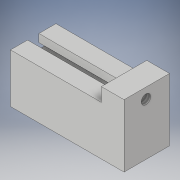
# Autodesk Inventor part: tenshoner base
Saved by Autodesk Inventor 2019 (Build 230136000, 136)
## iProperties
Created: 2019-12-07
Part Number: tenshoner base
Material: Generic
Document SubType Name: Modeling
Designer: User
Density: 1 g/cm^3
Appearance: Default
Author: User
Autodesk Inventor part; units mm, degrees
ref_plane "YZ Plane" through (0, 0, 0) normal (1, 0, 0) x (0, 1, 0)
ref_plane "XZ Plane" through (0, 0, 0) normal (0, 1, 0) x (-1, 0, 0)
ref_plane "XY Plane" through (0, 0, 0) normal (0, 0, 1) x (1, 0, 0)
sketch "Sketch1" plane through (0, 0, 0) normal (1, 0, 0) x (0, 1, 0)
  line L0 (0, 0) -> (13.716, 0)
  line L1 (13.716, 0) -> (13.716, -12.7)
  line L2 (13.716, -12.7) -> (0, -12.7)
  line L3 (0, -12.7) -> (0, 0)
  line L4 (13.716, -4.7625) -> (11.5062, -4.7625)
  line L5 (11.5062, -4.7625) -> (11.5062, -3.175)
  line L6 (11.5062, -3.175) -> (9.906, -3.175)
  line L7 (9.906, -3.175) -> (9.906, -9.525)
  line L8 (9.906, -9.525) -> (11.5062, -9.525)
  line L9 (11.5062, -9.525) -> (11.5062, -7.9375)
  line L10 (11.5062, -7.9375) -> (13.716, -7.9375)
  dimension "d0" = 12.7
  dimension "d1" = 3.175
  dimension "d2" = 6.35
  dimension "d3" = 1.5875
  dimension "d4" = 4.7625
  dimension "d5" = 1.6002
  dimension "d6" = 3.81
  dimension "d7" = 13.716
  constraints: 22 end point, 6 perpendicular, 4 point on line, 2 horizontal, 2 parallel
  measures "d0" distance of L0.end L1.end
  measures "d1" distance between parallel lines of L4 L10
  measures "d2" distance between parallel lines of L8 L6
  measures "d3" distance between parallel lines of L4 L6
  measures "d4" distance between parallel lines of L0 L4
  measures "d5" distance between parallel lines of L7 L5
  measures "d6" distance between parallel lines of L1 L7
  measures "d7" distance between parallel lines of L3 L1
extrude "Extrusion1" add sketch "Sketch1" along normal blind 25.4 contours L0 L1 L4 L5 L6 L7 L8 L9 L10 L2 L3
sketch "Sketch2" plane through (25.4, 0, 0) normal (1, 0, 0) x (0, 0, -1)
  line L0 (0, 0) -> (12.7, 0)
  line L1 (12.7, 0) -> (12.7, 17.526)
  line L2 (12.7, 17.526) -> (0, 17.526)
  line L3 (0, 17.526) -> (0, 0)
  line L4 (12.7, 13.716) -> (7.9375, 13.716) projected
  dimension "d10" = 3.81
  dimension "d11" = 12.7
  constraints: 8 end point, 2 parallel, 1 coincident, 1 horizontal, 1 perpendicular
  measures "d10" distance between parallel lines of L2 L4
  measures "d11" distance between parallel lines of L3 L1
extrude "Extrusion2" add sketch "Sketch2" along normal blind 6.35
sketch "Sketch3" plane through (31.75, 0, 0) normal (1, 0, 0) x (0, 0, -1)
  line L0 (0, 0) -> (12.7, 0) projected
  line L1 (12.7, 0) -> (12.7, 17.526) projected
  line L2 (12.7, 17.526) -> (0, 17.526) projected
  line L3 (0, 17.526) -> (0, 0) projected
  line L4 (0, 0) -> (12.7, 0) projected
  line L5 (0, 13.716) -> (0, 0) projected
  line L6 (4.7625, 13.716) -> (0, 13.716) projected
  line L7 (4.7625, 11.5062) -> (4.7625, 13.716) projected
  line L8 (3.175, 11.5062) -> (4.7625, 11.5062) projected
  line L9 (3.175, 9.906) -> (3.175, 11.5062) projected
  line L10 (9.525, 9.906) -> (3.175, 9.906) projected
  line L11 (9.525, 11.5062) -> (9.525, 9.906) projected
  line L12 (7.9375, 11.5062) -> (9.525, 11.5062) projected
  line L13 (7.9375, 13.716) -> (7.9375, 11.5062) projected
  line L14 (12.7, 13.716) -> (7.9375, 13.716) projected
  line L15 (12.7, 0) -> (12.7, 13.716) projected
  line L16 (0, 0) -> (12.7, 0) projected
  line L17 (0, 13.716) -> (0, 0) projected
  line L18 (4.7625, 13.716) -> (0, 13.716) projected
  line L19 (4.7625, 11.5062) -> (4.7625, 13.716) projected
  line L20 (3.175, 11.5062) -> (4.7625, 11.5062) projected
  line L21 (3.175, 9.906) -> (3.175, 11.5062) projected
  line L22 (9.525, 9.906) -> (3.175, 9.906) projected
  line L23 (9.525, 11.5062) -> (9.525, 9.906) projected
  line L24 (7.9375, 11.5062) -> (9.525, 11.5062) projected
  line L25 (7.9375, 13.716) -> (7.9375, 11.5062) projected
  line L26 (12.7, 13.716) -> (7.9375, 13.716) projected
  line L27 (12.7, 0) -> (12.7, 13.716) projected
  line L28 (4.7625, 13.716) -> (0, 13.716) projected
  line L29 (9.525, 9.906) -> (3.175, 9.906) projected
  line L30 (0, 0) -> (12.7, 0) projected
  line L31 (0, 13.716) -> (0, 0) projected
  line L32 (4.7625, 13.716) -> (0, 13.716) projected
  line L33 (4.7625, 11.5062) -> (4.7625, 13.716) projected
  line L34 (3.175, 11.5062) -> (4.7625, 11.5062) projected
  line L35 (3.175, 9.906) -> (3.175, 11.5062) projected
  line L36 (9.525, 9.906) -> (3.175, 9.906) projected
  line L37 (9.525, 11.5062) -> (9.525, 9.906) projected
  line L38 (7.9375, 11.5062) -> (9.525, 11.5062) projected
  line L39 (7.9375, 13.716) -> (7.9375, 11.5062) projected
  line L40 (12.7, 13.716) -> (7.9375, 13.716) projected
  line L41 (12.7, 0) -> (12.7, 13.716) projected
  point P0 (6.1226, 14.5707)
hole "Hole1" at (31.75, 14.5707, -6.1226) direction (-1, 0, 0) diameter 2.6416 depth 6.35 tip angle 118 thread size "6-32 UNC" class "2B" standard "ANSI Unified Screw Threads"
equation "\"d3\" = -0.5 * d1 + 0.5 * d2"
equation "\"d4\" = -0.5 * d1 + 0.5 * d0"
body "Solid1"
